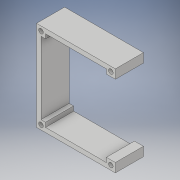
# Autodesk Inventor part: Gearbox cover
Saved by Autodesk Inventor 2018 (Build 220112000, 112)
## iProperties
Created: 2019-01-19
Part Number: Gearbox cover
Material: Generic
Document SubType Name: Modeling
Designer: maste
Density: 1 g/cm^3
Appearance: Default
Author: maste
Autodesk Inventor part; units mm, degrees
ref_plane "YZ Plane" through (0, 0, 0) normal (1, 0, 0) x (0, 1, 0)
ref_plane "XZ Plane" through (0, 0, 0) normal (0, 1, 0) x (-1, 0, 0)
ref_plane "XY Plane" through (0, 0, 0) normal (0, 0, 1) x (1, 0, 0)
sketch "Sketch1" plane through (0, 0, 0) normal (0, 0, 1) x (1, 0, 0)
  line L0 (0, 0) -> (0, 101.6)
  line L1 (0, 101.6) -> (88.9, 101.6)
  line L2 (0, 0) -> (88.9, 0)
  arc A0 (88.9, 0) -> (88.9, 101.6) centre (-27.4974, 50.8) ccw
  line L3 (0, 101.6) -> (5.08, 101.6) construction
  line L4 (5.08, 101.6) -> (5.08, 96.52) construction
  circle A1 centre (5.08, 96.52) radius 2.5797
  line L5 (44.45, 101.6) -> (44.45, 0) construction
  line L6 (0, 50.8) -> (104.3223, 50.8) construction
  circle A2 centre (83.82, 96.52) radius 2.5797
  circle A3 centre (5.08, 5.08) radius 2.5797
  circle A4 centre (83.82, 5.08) radius 2.5797
  line L7 (0, 101.6) -> (10.16, 101.6) construction
  line L8 (0, 101.6) -> (0, 91.44) construction
  line L9 (10.16, 96.52) -> (10.16, 91.44)
  line L10 (10.16, 91.44) -> (5.08, 91.44)
  line L11 (5.08, 91.44) -> (5.08, 50.8)
  line L12 (10.16, 96.52) -> (44.45, 96.52)
  arc A5 (90.1405, 10.16) -> (90.1405, 91.44) centre (-27.4974, 50.8) ccw
  line L13 (84.2708, 99.06) -> (83.3692, 99.06)
  line L14 (78.74, 96.52) -> (78.74, 91.44)
  line L15 (78.74, 91.44) -> (90.1405, 91.44)
  line L16 (78.74, 96.52) -> (44.45, 96.52)
  line L17 (10.16, 5.08) -> (10.16, 10.16)
  line L18 (10.16, 10.16) -> (5.08, 10.16)
  line L19 (10.16, 5.08) -> (44.45, 5.08)
  line L20 (78.74, 5.08) -> (44.45, 5.08)
  line L21 (78.74, 5.08) -> (78.74, 10.16)
  line L22 (78.74, 10.16) -> (90.1405, 10.16)
  line L23 (5.08, 10.16) -> (5.08, 50.8)
  point P0 (78.74, 101.6)
  point P1 (88.9, 91.44)
  point P2 (10.16, 0)
  point P3 (0, 10.16)
  point P4 (78.74, 0)
  point P5 (88.9, 10.16)
  dimension "d0" = 101.6
  dimension "d1" = 88.9
  dimension "d2" = 88.9
  dimension "d3" = 127
  dimension "d4" = 5.08
  dimension "d5" = 5.08
  dimension "d6" = 5.1594
  dimension "d7" = 10.16
  dimension "d8" = 10.16
  dimension "d9" = 2.54
  constraints: 48 end point, 17 symmetric about line, 7 point on line, 6 centre point, 6 point on circle, 5 perpendicular, 3 midpoint, 2 horizontal, 2 vertical, 1 coincident, 3 other
  measures "d0" distance of L0.start L0.end
  measures "d1" distance of L0.end L1.end
  measures "d2" distance of L0.start L2.end
  measures "d3" radius of A0
  measures "d4" distance of L0.end L3.end
  measures "d5" distance of L3.end L4.end
  measures "d6" diameter of A1
  measures "d7" distance of L0.end L7.end
  measures "d8" distance of L0.end L8.end
  measures "d9" radial gap between concentric circles of A0 A5
extrude "Extrusion1" add sketch "Sketch1" along normal blind 31.6992
sketch "Sketch2" plane through (0, 0, 31.6992) normal (0, 0, 1) x (1, 0, 0)
  line L0 (88.9, 0) -> (0, 0) projected
  line L1 (88.9, 0) -> (124.549, 0)
  line L2 (124.549, 0) -> (124.549, 101.6)
  line L3 (124.549, 101.6) -> (88.9, 101.6)
  line L4 (88.9, 101.6) -> (88.9, 0)
  constraints: 8 end point, 2 parallel, 1 horizontal, 1 perpendicular
extrude "Extrusion2" cut sketch "Sketch2" against normal blind 31.6992
body "Solid1"
